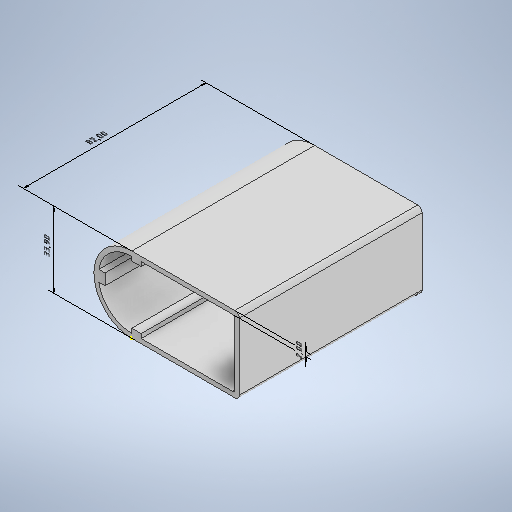
# Autodesk Inventor part: schranka
Saved by Autodesk Inventor 2025.3 (Build 293356000, 356)
## iProperties
Created: 2025-06-12
Part Number: schranka
Material: Generic
Document SubType Name: Modeling
Designer: Repete
Density: 1 g/cm^3
Appearance: Default
Author: Repete
Autodesk Inventor part; units mm, degrees
ref_plane "YZ Plane" through (0, 0, 0) normal (1, 0, 0) x (0, 1, 0)
ref_plane "XZ Plane" through (0, 0, 0) normal (0, 1, 0) x (-1, 0, 0)
ref_plane "XY Plane" through (0, 0, 0) normal (0, 0, 1) x (1, 0, 0)
sketch "Sketch1" plane through (0, 0, 0) normal (0, 1, 0) x (-1, 0, 0)
  line L0 (-15.6488, -14.9) -> (-4.1777, -14.9)
  line L1 (-4.1777, 15) -> (-13.2013, 15)
  line L2 (14.7902, 2.5) -> (12, 2.5)
  line L3 (12, 2.5) -> (12, -2.5)
  line L4 (12, -2.5) -> (14.7902, -2.5)
  arc A0 (0, -15) -> (14.7902, -2.5) centre (0, 0) ccw
  arc A1 (14.7902, 2.5) -> (0, 15) centre (0, 0) ccw
  line L5 (0.0236, 15) -> (0.0236, 15.0064)
  line L6 (0.0236, 13.1) -> (-4.1777, 13.1)
  line L7 (-4.1777, 13.1) -> (-4.1777, 15)
  line L8 (-0.1777, -13) -> (-4.1777, -13)
  line L9 (-4.1777, -13) -> (0, -13)
  line L10 (-4.1777, -14.9) -> (-4.1777, -13)
  line L11 (-13.2013, 15) -> (-46.2013, 15)
  line L12 (-15.6488, -14.9) -> (-46.2013, -14.9)
  line L13 (-46.2013, -14.9) -> (-46.2013, 15)
  arc A2 (-1.8412, -16.9) -> (0, 17) centre (0, 0) ccw
  line L14 (0, 17) -> (-48.2013, 17)
  line L15 (-48.2013, 17) -> (-48.2013, -16.9)
  line L16 (-48.2013, -16.9) -> (-1.8412, -16.9)
  line L17 (0.0236, 15) -> (0.0236, 13.1)
  line L18 (0, -13) -> (0, -15)
  point P0 (-13.2013, 0)
  point P1 (12.5, 0)
  point P2 (11.0065, 21.7068)
  point P3 (11.0065, 50.7004)
  dimension "d0" = 30
  dimension "d7" = 33
  dimension "d8" = 2
  dimension "d9" = 2
  dimension "d10" = 2
  dimension "d11" = 2
  dimension "d34" = 1.9
  dimension "d35" = 1.9
  dimension "d36" = 10.5
  dimension "d37" = 5
  dimension "d38" = 12
  dimension "d39" = 15
  constraints: 38 end point, 7 point on circle, 5 horizontal, 4 parallel, 4 perpendicular, 3 centre point, 1 coincident, 1 vertical
  measures "d0" distance of L1.end L0.start
  measures "d7" distance from line of L13 point (-13.201, 0)
  measures "d8" radial gap between concentric circles of A0 A2
  measures "d9" distance between parallel lines of L15 L13
  measures "d10" distance between parallel lines of L0 L16
  measures "d11" distance between parallel lines of L14 L11
  measures "d34" distance between parallel lines of L1 L6
  measures "d35" distance between parallel lines of L0 L8
  measures "d36" distance between parallel lines of L8 L4
  measures "d37" distance of L2.end L3.end
  measures "d38" distance from line of A0.centre L3
  measures "d39" radius of A1
extrude "Extrusion1" add sketch "Sketch1" along normal blind 80
ref_plane "Work Plane1" through (0, 82, 0) normal (0, 1, 0) x (1, 0, 0)
sketch "Sketch3" plane through (0, 82, 0) normal (0, 1, 0) x (1, 0, 0)
  arc A0 (0, 17) -> (0, -17) centre (0, 0) ccw
  line L0 (0, -17) -> (48.2013, -17)
  line L1 (48.2013, -17) -> (48.2013, 17)
  line L2 (48.2013, 17) -> (0, 17)
  point P0 (13.2013, 0)
  point P1 (-14.9845, -166.3883)
  point P2 (-14.9845, -137.3947)
  point P3 (-26.1687, -202.0885)
  constraints: 6 end point, 2 point on circle, 1 centre point, 1 parallel, 1 perpendicular
extrude "Extrusion2" add sketch "Sketch3" against normal up to surface (2 mm away)
sketch "Sketch4" plane through (48.2013, 0, -16.9) normal (0, 0, -1) x (-1, 0, 0)
  point P0 (48.2013, 0)
fillet "Fillet1" radius 2 2 edges at (48.2013, 40, -16.9) (48.2013, 41, 17)
fillet "Fillet2" radius 1 2 edges at (46.2013, 40, 15) (46.2013, 40, -14.9)
fillet "Fillet3" radius 2 1 edges at (48.2013, 81, -17)
body "Solid1"
